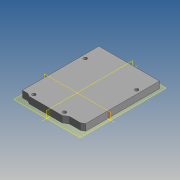
# Autodesk Inventor part: P016_FondBoitierCapteurs
Saved by Autodesk Inventor 2021.3 (Build 253353000, 353)
## iProperties
Created: 2021-10-29
Part Number: P016_FondBoitierCapteurs
Material: Générique
Document SubType Name: Modeling
Designer: gabri
Density: 1 g/cm^3
Appearance: Par défaut
Author: gabri
Autodesk Inventor part; units mm, degrees
sketch "Sketch2" plane through (0, 0, 0) normal (0, 0, 1) x (1, 0, 0)
  line L0 (-19.3634, -24.3013) -> (10.6366, -24.3013)
  line L1 (27.9921, -20.0546) -> (27.9921, 47.2987)
  line L2 (27.9921, 47.2987) -> (-27.3079, 47.2987)
  line L3 (-27.3079, 47.2987) -> (-27.3079, -22.6013)
  line L4 (-27.4978, -24.3206) -> (27.9921, 47.2987) construction
  line L5 (27.3079, -47.2987) -> (-27.3079, 47.2987) construction
  line L6 (-27.3079, -22.6013) -> (-22.3079, -22.6013)
  line L7 (-22.3079, -22.6013) -> (-19.3634, -24.3013)
  line L8 (27.9921, -20.0546) -> (24.9667, -21.8013)
  line L9 (24.9667, -21.8013) -> (14.9667, -21.8013)
  line L10 (14.9667, -21.8013) -> (10.6366, -24.3013)
  point P0 (-3.6954, 6.4006)
  point P1 (0, 0)
  point P2 (0, 0)
  dimension "d24" = 55.3
  dimension "d25" = 71.6
  dimension "d26" = 69.9
  dimension "d27" = 5
  dimension "d28" = 150
  dimension "d29" = 150
  dimension "d30" = 69.1
  dimension "d31" = 10
  dimension "d32" = 30
  dimension "d33" = 120
  dimension "d34" = 37.768
  dimension "d35" = 27.9921
  dimension "d36" = 55.4899
  constraints: 22 end point, 3 parallel, 2 horizontal, 2 perpendicular, 2 point on line, 1 coincident, 1 midpoint
  measures "d24" distance of L1.end L2.end
  measures "d25" distance between parallel lines of L0 L2
  measures "d26" distance between parallel lines of L2 L6
  measures "d27" distance of L3.end L6.end
  measures "d28" angle of L6 L7
  measures "d29" angle of L10 L9
  measures "d30" distance between parallel lines of L2 L9
  measures "d31" distance of L8.end L9.end
  measures "d32" distance of L0.start L0.end
  measures "d33" angle of L8 L1
  measures "d34" angle of L4 L1
  measures "d35" distance from line of point (0, 0) L1
  measures "d36" distance from line of L4.start L1
extrude "Extrusion1" add sketch "Sketch2" along normal blind 6
sketch "Sketch3" plane through (0, 0, 6) normal (0, 0, 1) x (1, 0, 0)
  line L0 (27.9921, 47.2987) -> (-27.3079, 47.2987) construction
  line L1 (-27.3079, 47.2987) -> (-27.3079, -22.6013) construction
  line L2 (-27.3079, -22.6013) -> (-22.3079, -22.6013) construction
  line L3 (-22.3079, -22.6013) -> (-19.3634, -24.3013) construction
  line L4 (-19.3634, -24.3013) -> (10.6366, -24.3013) construction
  line L5 (10.6366, -24.3013) -> (14.9667, -21.8013) construction
  line L6 (14.9667, -21.8013) -> (24.9667, -21.8013) construction
  line L7 (24.9667, -21.8013) -> (27.9921, -20.0546) construction
  line L8 (27.9921, -20.0546) -> (27.9921, 47.2987) construction
  point P0 (0, 0)
  point P1 (24.3921, 29.9987)
  point P2 (-23.8079, 31.2987)
  point P3 (-18.7079, -20.8013)
  point P4 (9.1921, -20.8013)
  dimension "d37" = 3.5
  dimension "d38" = 16
  dimension "d39" = 48.2
  dimension "d40" = 55.3
  dimension "d42" = 17.3
  dimension "d43" = 50.8
  dimension "d44" = 52.1
  dimension "d45" = 27.9
  dimension "d46" = 8.6
  measures "d37" distance from line of L1 point (-23.808, 31.299)
  measures "d38" distance from line of L0 point (-23.808, 31.299)
  measures "d39" horizontal distance of point (24.392, 29.999) point (-23.808, 31.299)
  measures "d40" distance of L0.start L0.end
  measures "d42" distance from line of L0 point (24.392, 29.999)
  measures "d43" vertical distance of point (9.192, -20.801) point (24.392, 29.999)
  measures "d44" vertical distance of point (-18.708, -20.801) point (-23.808, 31.299)
  measures "d45" distance of point (-18.708, -20.801) point (9.192, -20.801)
  measures "d46" distance from line of L1 point (-18.708, -20.801)
hole "Hole1" at (9.1921, -20.8013, 6) at (24.3921, 29.9987, 6) at (-23.8079, 31.2987, 6) at (-18.7079, -20.8013, 6) direction (0, 0, -1) diameter 3.1 depth 6 tip angle 118
body "Solid1"
